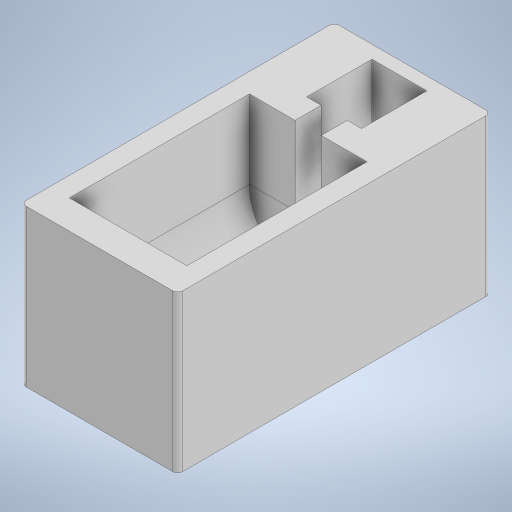
# Autodesk Inventor part: housing_V2
Saved by Autodesk Inventor 2023 (Build 270158000, 158)
## iProperties
Created: 2023-03-23
Part Number: housing_V2
Material: Generic
Document SubType Name: Modeling
Designer: caleb
Density: 1 g/cm^3
Appearance: Default
Author: caleb
## iProperties of the stored document housing_V2_3DPrint.ipt
Created: 2023-03-24
Part Number: housing_V2_3DPrint
Material: Generic
Document SubType Name: Modeling
Designer: caleb
Density: 1 g/cm^3
Appearance: Default
Author: caleb
Autodesk Inventor part; units mm, degrees
sketch "Sketch1" plane through (0, 0, 0) normal (0, 1, 0) x (-1, 0, 0)
  line L0 (-0.0661, 0.1517) -> (59.9339, 0.1517)
  line L1 (59.9339, 0.1517) -> (59.9339, -119.8483)
  line L2 (59.9339, -119.8483) -> (-0.0661, -119.8483)
  line L3 (-0.0661, -119.8483) -> (-0.0661, 0.1517)
  line L4 (29.9339, -119.8483) -> (29.9339, 0.1517)
  circle A0 centre (29.9339, -54.8547) radius 22.5
  line L5 (19.5008, -89.8484) -> (19.5008, -114.8484)
  line L6 (19.5008, -114.8484) -> (40.5008, -114.8484)
  line L7 (40.5008, -114.8484) -> (40.5008, -89.8484)
  line L8 (40.5008, -89.8484) -> (19.5008, -89.8484)
  line L9 (19.5008, -89.8484) -> (40.5008, -114.8484) construction
  line L10 (19.5008, -114.8484) -> (40.5008, -89.8484) construction
  line L11 (19.5008, -89.8484) -> (44.5008, -89.8484) construction
  line L12 (24.9546, -79.8533) -> (24.9546, -89.8533)
  line L13 (24.9546, -89.8533) -> (34.9546, -89.8533)
  line L14 (34.9546, -89.8533) -> (34.9546, -79.8533)
  line L15 (34.9546, -79.8533) -> (24.9546, -79.8533)
  line L16 (24.9546, -79.8533) -> (34.9546, -89.8533) construction
  line L17 (24.9546, -89.8533) -> (34.9546, -79.8533) construction
  line L18 (24.9546, -79.8533) -> (34.9546, -79.8533) construction
  line L19 (7.4339, -10.8533) -> (7.4339, -79.8533)
  line L20 (7.4339, -79.8533) -> (52.4339, -79.8533)
  line L21 (52.4339, -79.8533) -> (52.4339, -10.8533)
  line L22 (52.4339, -10.8533) -> (7.4339, -10.8533)
  line L23 (7.4339, -10.8533) -> (52.4339, -79.8533) construction
  line L24 (7.4339, -79.8533) -> (52.4339, -10.8533) construction
  line L25 (7.4339, -10.8533) -> (76.4339, -10.8533) construction
  line L26 (34.9339, -5.8533) -> (24.9339, -5.8533)
  line L27 (24.9339, -5.8533) -> (24.9339, -15.8533)
  line L28 (24.9339, -15.8533) -> (34.9339, -15.8533)
  line L29 (34.9339, -15.8533) -> (34.9339, -5.8533)
  line L30 (34.9339, -5.8533) -> (24.9339, -15.8533) construction
  line L31 (24.9339, -5.8533) -> (34.9339, -15.8533) construction
  point P0 (0, 0)
  point P1 (29.9339, -114.8483)
  point P2 (30.4342, -89.8533)
  point P3 (29.9546, -89.8533)
  point P4 (29.9339, -79.8533)
  point P5 (30.0136, -77.3546)
  point P6 (29.9339, -25)
  point P7 (30.0008, -102.3484)
  point P8 (29.9339, -10.8533)
  point P9 (29.9546, -84.8533)
  point P10 (29.9339, -10.8533)
  point P11 (29.9339, -45.3533)
  point P12 (34.9546, -79.8533)
  point P13 (24.9546, -79.8533)
  point P14 (24.9546, -89.8484)
  point P15 (34.9546, -89.8484)
  point P16 (34.9339, -10.8533)
  point P17 (24.9339, -10.8533)
  dimension "d0" = 60
  dimension "d1" = 120
  dimension "d2" = 45
  dimension "d3" = 5
  dimension "d4" = 25
  dimension "d6" = 12.5
  dimension "d7" = 10
  dimension "d8" = 2.5
  dimension "d9" = 22.5
  dimension "d10" = -69
  dimension "d11" = 25
  dimension "d12" = 90
  dimension "d13" = 21
  dimension "d14" = 5
  dimension "d15" = 10
  dimension "d16" = 90
  dimension "d17" = 10
  dimension "d18" = -69
  dimension "d19" = 90
  dimension "d20" = -34.5
  dimension "d21" = 45
  dimension "d42" = 10
  dimension "d43" = 10
  constraints: 64 end point, 13 parallel, 11 midpoint, 8 perpendicular, 6 point on line, 4 horizontal, 2 coincident, 1 centre point
  measures "d0" distance of L2.start L2.end
  measures "d1" distance of L1.start L2.start
  measures "d2" diameter of A0
  measures "d3" distance from line of L2 point (29.934, -114.848)
  measures "d4" distance of point (30.434, -89.853) point (29.934, -114.848)
  measures "d6" distance of point (29.934, -114.848) point (30.001, -102.348)
  measures "d7" distance of point (29.934, -79.853) point (29.955, -89.853)
  measures "d8" distance of point (30.014, -77.355) point (29.934, -79.853)
  measures "d9" distance of point (29.934, -54.855) point (30.014, -77.355)
  measures "d10" distance of point (29.934, -10.853) point (29.934, -79.853)
  measures "d11" distance of L8.end L5.end
  measures "d12" angle of L5 L11
  measures "d13" distance of L7.start L5.end
  measures "d14" distance of point (29.955, -84.853) point (29.955, -89.853)
  measures "d15" distance of L15.end L12.end
  measures "d16" angle of L12 L18
  measures "d17" distance of L14.start L12.end
  measures "d18" distance of L19.start L20.start
  measures "d19" angle of L19 L25
  measures "d20" distance of point (29.934, -79.853) point (29.934, -45.353)
  measures "d21" distance between parallel lines of L19 L21
  measures "d42" distance of L26.start L26.end
  measures "d43" distance of L27.end L26.end
extrude "Extrusion1" add sketch "Sketch1" against normal blind 60
sketch "Sketch2" plane through (0.0661, 0, -119.8483) normal (0, 0, -1) x (-1, 0, 0)
  line L0 (0, 0) -> (60, 0) projected
  line L1 (0, 0) -> (0, -60) projected
  line L2 (60, -60) -> (0, -60) projected
  line L3 (60, 0) -> (60, -60) projected
  point P0 (0.0661, 0)
  point P1 (30, -30)
ref_plane "Work Plane1" through (-19.5008, 0, -114.8484) normal (0, 0, -1) x (-1, 0, 0)
ref_plane "Work Plane2" through (-19.5008, 0, -89.8484) normal (0, 0, -1) x (-1, 0, 0)
ref_plane "Work Plane3" through (-24.9546, 0, -79.8533) normal (0, 0, -1) x (-1, 0, 0)
ref_plane "Work Plane5" through (-7.4339, 0, -5.8533) normal (0, 0, -1) x (-1, 0, 0)
ref_plane "Work Plane4" through (-7.4339, 0, -10.8533) normal (0, 0, -1) x (-1, 0, 0)
sketch "Sketch3" plane through (-19.5008, 0, -114.8484) normal (0, 0, -1) x (-1, 0, 0)
  circle A0 centre (10.433, -30) radius 10.5
  point P0 (-19.5008, 0)
  dimension "d25" = 21
  constraints: 1 centre point, 1 coincident
  measures "d25" diameter of A0
ref_plane "Work Plane6" through (-29.9339, -30, -119.8483) normal (0, 1, 0) x (1, 0, 0)
extrude "Extrusion3" cut sketch "Sketch1" against normal up to surface (30 mm away) contours L22 L29 L28 L4 | L4 L28 L27 L22 | L6 L5 L8 L12 L13 L4 | L4 L13 L14 L8 L7 L6 | L28 L29 L22 L21 A0 L4 | L4 A0 L19 L22 L27 L28 | L13 L12 L8 L4 | L4 L8 L14 L13 | A0 L4 | L4 A0 | L8 L12 L15 L4 | L4 L15 L14 L8 | A0 L21 L20 L15 L4 | L4 L15 L20 L19 A0
sketch "Sketch4" plane through (-19.5008, 0, -89.8484) normal (0, 0, -1) x (-1, 0, 0)
  circle A0 centre (10.433, -30) radius 5
  point P0 (-19.5008, 0)
  point P1 (15.4537, 0)
  point P2 (15.4537, 0)
  point P3 (15.4537, 0)
  point P4 (5.4537, 0)
  point P5 (5.4537, 0)
  point P6 (5.4537, 0)
  dimension "d30" = 10
  constraints: 1 centre point, 1 coincident
  measures "d30" diameter of A0
sketch "Sketch5" plane through (-24.9546, 0, -79.8533) normal (0, 0, -1) x (-1, 0, 0)
  circle A0 centre (4.9793, -30) radius 22.5
  point P0 (-24.9546, 0)
  dimension "d31" = 45
  constraints: 1 centre point, 1 coincident
  measures "d31" diameter of A0
extrude "Extrusion4" cut sketch "Sketch3" against normal up to surface (25 mm away)
ref_plane "Work Plane7" through (0.0661, 0, -117.8483) normal (0, 0, -1) x (-1, 0, 0)
extrude "Extrusion5" cut sketch "Sketch4" against normal up to surface (83.9952 mm away)
extrude "Extrusion6" cut sketch "Sketch5" against normal up to surface (69 mm away)
extrude "Extrusion7" cut sketch "Sketch4" along normal up to surface (27.9998 mm away)
fillet "Fillet1" radius 2 4 edges at (-59.9339, -30, 0.1517) (0.0661, -30, 0.1517) (0.0661, -30, -119.8483) (-59.9339, -30, -119.8483)
extrude "Extrusion8" cut sketch "Sketch1" against normal through all contours L22 L29 L28 L4 | L4 L28 L27 L22
chamfer "Chamfer1" distance 2 angle 45 4 edges at (-29.9339, -60, -10.8533) (-24.9339, -60, -13.3533) (-29.9339, -60, -15.8533) (-34.9339, -60, -13.3533)
chamfer "Chamfer2" distance 2 angle 45 3 edges at (-34.9339, -51.9374, -13.3533) (-29.9339, -52.5, -15.8533) (-24.9339, -51.9374, -13.3533)
fillet "Fillet2" radius 1 1 edges at (-24.9339, -30, -114.8484)
fillet "Fillet3" radius 1 1 edges at (-24.9339, -30, -10.8533)
sketch "Sketch6" plane through (0, -60, 0) normal (0, -1, 0) x (1, 0, 0)
  arc A0 (-59.9339, -117.8483) -> (-57.9339, -119.8483) centre (-57.9339, -117.8483) ccw projected
  line L0 (-57.9339, -119.8483) -> (-1.9339, -119.8483) projected
  arc A1 (-1.9339, -119.8483) -> (0.0661, -117.8483) centre (-1.9339, -117.8483) ccw projected
  line L1 (0.0661, -117.8483) -> (0.0661, -1.8483) projected
  arc A2 (0.0661, -1.8483) -> (-1.9339, 0.1517) centre (-1.9339, -1.8483) ccw projected
  line L2 (-1.9339, 0.1517) -> (-57.9339, 0.1517) projected
  arc A3 (-57.9339, 0.1517) -> (-59.9339, -1.8483) centre (-57.9339, -1.8483) ccw projected
  line L3 (-59.9339, -1.8483) -> (-59.9339, -117.8483) projected
  line L4 (-36.9339, -8.8533) -> (-36.9339, -17.8533) projected
  line L5 (-22.9339, -8.8533) -> (-36.9339, -8.8533) projected
  line L6 (-22.9339, -17.8533) -> (-22.9339, -8.8533) projected
  line L7 (-36.9339, -17.8533) -> (-22.9339, -17.8533) projected
  line L8 (-29.9339, 0.1517) -> (-29.9339, -119.8483)
  line L9 (0.0661, -59.8483) -> (-59.9339, -59.8483)
  line L10 (-29.9339, -59.8483) -> (-29.9339, -119.8483)
  line L11 (-29.9339, -59.8483) -> (-29.9339, -89.8483)
  line L12 (-29.9339, -89.8483) -> (-29.9339, -119.8483)
  line L13 (-29.9339, -89.8483) -> (-59.9339, -89.8483)
  line L14 (-59.9339, -89.8483) -> (-59.9339, -119.8483)
  line L15 (-59.9339, -119.8483) -> (-29.9339, -119.8483)
  line L16 (-29.9339, -119.8483) -> (-29.9339, -89.8483)
  circle A4 centre (-44.9339, -104.8483) radius 3.75
  circle A5 centre (-14.9339, -104.8483) radius 3.75
  circle A6 centre (-44.9339, -74.8483) radius 3.75
  circle A7 centre (-14.9339, -74.8483) radius 3.75
  point P0 (0, 0)
  point P1 (-29.9339, -74.8483)
  point P2 (-29.9339, -104.8483)
  dimension "d58" = 7.5
  dimension "d61" = 30
  dimension "d64" = 30
  constraints: 18 end point, 8 midpoint, 4 centre point, 4 coincident, 3 equal length, 2 horizontal, 2 perpendicular, 1 vertical, 9 other
  measures "d58" diameter of A4
  measures "d61" distance of A4.centre A5.centre
  measures "d64" distance of A4.centre A6.centre
extrude "Extrusion10" add sketch "Sketch6" along normal blind 5 contours A4 | A5 | A6 | A7
equation "\"d4\" = d11"
equation "\"d6\" = 0.5 * d4"
equation "\"d7\" = d15"
equation "\"d9\" = 0.5 * d2"
equation "\"d14\" = 0.5 * d7"
equation "\"d18\" = d10"
equation "\"d20\" = 0.5 * d10"
equation "\"d21\" = d2"
equation "\"d31\" = d2"
body "Solid1"
